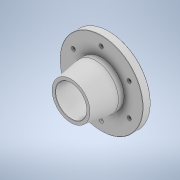
# Autodesk Inventor part: ExtendedIndexerPivot
Saved by Autodesk Inventor 2020 (Build 240168000, 168)
## iProperties
Created: 2020-01-29
Part Number: ExtendedIndexerPivot
Material: Generic
Document SubType Name: Modeling
Designer: srini
Density: 1 g/cm^3
Appearance: Default
Author: srini
Autodesk Inventor part; units mm, degrees
ref_plane "YZ Plane" through (0, 0, 0) normal (1, 0, 0) x (0, 1, 0)
ref_plane "XZ Plane" through (0, 0, 0) normal (0, 1, 0) x (-1, 0, 0)
ref_plane "XY Plane" through (0, 0, 0) normal (0, 0, 1) x (1, 0, 0)
sketch "Sketch1" plane through (0, 0, 0) normal (0, 0, 1) x (1, 0, 0)
  circle A0 centre (0, 0) radius 26.054
  circle A1 centre (0, 0) radius 69.55
  circle A2 centre (0, 53.975) radius 3.3734
  circle A3 centre (-46.7437, 26.9875) radius 3.3734
  circle A4 centre (-46.7437, -26.9875) radius 3.3734
  circle A5 centre (0, -53.975) radius 3.3734
  circle A6 centre (46.7437, -26.9875) radius 3.3734
  circle A7 centre (46.7437, 26.9875) radius 3.3734
  dimension "d0" = 52.108
  dimension "d1" = 139.1
  dimension "d2" = 6.7469
  dimension "d3" = 53.975
  dimension "d6" = 360
  constraints: 8 centre point, 2 coincident, 1 vertical alignment, 13 other
  measures "d0" diameter of A0
  measures "d1" diameter of A1
  measures "d2" diameter of A2
  measures "d3" distance of point (0, 0) A2.centre
extrude "Extrusion1" add sketch "Sketch1" along normal blind 12.7
sketch "Sketch2" plane through (0, 0, 12.7) normal (0, 0, 1) x (1, 0, 0)
  circle A0 centre (0, 0) radius 38.1
  circle A1 centre (0, 0) radius 26.054 projected
  dimension "d10" = 76.2
  constraints: 1 centre point, 1 coincident
  measures "d10" diameter of A0
extrude "Extrusion2" add sketch "Sketch2" along normal blind 50.8
chamfer "Chamfer1" distance 6.35 distance2 41.275 1 edges at (-38.1, 0, 63.5) measured on face at (33.7663, -2.826, 63.5)
chamfer "Chamfer2" distance 0.508 angle 45 4 edges at (-69.55, 0, 12.7) (-69.55, 0, 0) (-26.054, 0, 0) (-26.054, 0, 63.5)
body "Solid1"
